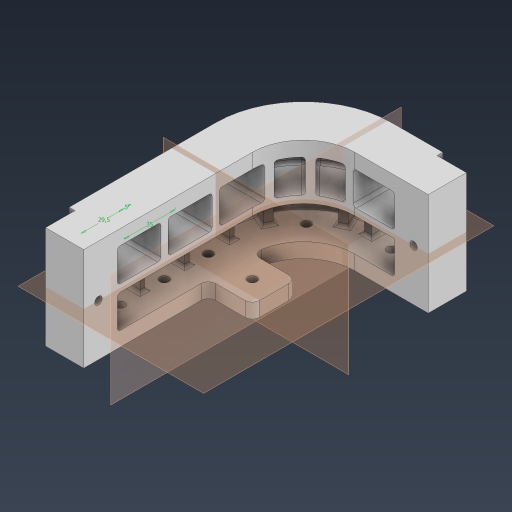
# Autodesk Inventor part: Верхняя часть столба зада
Saved by Autodesk Inventor 2023.2 (Build 272271030, 271C)
## iProperties
Created: 2025-09-30
Part Number: Верхняя часть столба зада
Material: Типовые
Document SubType Name: Modeling
Designer: Олег Коноваленко
Density: 1 g/cm^3
Appearance: По умолчанию
Author: Олег Коноваленко
Autodesk Inventor part; units mm, degrees
sketch "Эскиз1" plane through (0, 0, 0) normal (0, 1, 0) x (-1, 0, 0)
  line L0 (57.5, -90) -> (57.5, 90)
  line L1 (57.5, 90) -> (27.5, 90)
  line L2 (27.5, 90) -> (27.5, -60)
  line L3 (27.5, -60) -> (-57.5, -60)
  line L4 (-57.5, -60) -> (-57.5, -90)
  line L5 (-57.5, -90) -> (57.5, -90)
  line L6 (27.5, 90) -> (-57.5, 90) construction
  line L7 (-57.5, 90) -> (-57.5, -60) construction
  line L8 (57.5, -90) -> (-57.5, 90) construction
  line L9 (-57.5, -90) -> (57.5, 90) construction
  arc A0 (-2.5, -90) -> (57.5, -30) centre (-2.5, -30) ccw
  arc A1 (-7.5, -60) -> (27.5, -25) centre (-7.5, -25) ccw
  point P0 (0, 0)
  point P1 (0, 0)
  dimension "d0" = 115
  dimension "d1" = 180
  dimension "d2" = 30
  dimension "d3" = 30
  dimension "d5" = 70
  dimension "d6" = 60
  constraints: 20 end point, 6 perpendicular, 4 point on circle, 4 point on line, 4 tangent, 2 centre point, 1 coincident, 1 horizontal, 1 midpoint, 1 vertical
  measures "d0" distance of L4.end L0.start
  measures "d1" distance of L0.start L0.end
  measures "d2" distance of L3.end L4.end
  measures "d3" distance of L0.end L1.end
  measures "d5" diameter of A1
  measures "d6" radius of A0
extrude "Выдавливание1" add sketch "Эскиз1" along normal mid plane 70 contours A0 L5 L4 L3 L2 L1 L0 | L2 L3 A1
shell "Оболочка1" thickness 5 removed faces 3 at (-25.0806, 11.6667, -37.7869) at (24.1667, 11.6667, -60) at (-27.5, 11.6667, 13.3333)
sketch "Эскиз2" plane through (0, 0, 0) normal (0, 1, 0) x (-1, 0, 0)
  line L0 (27.5, -25) -> (27.5, 85) projected
  arc A0 (-7.5, -60) -> (27.5, -25) centre (-7.5, -25) ccw projected
  line L1 (-52.5, -60) -> (-7.5, -60) projected
  line L2 (-52.5, -85) -> (-52.5, -60) projected
  line L3 (-2.5, -85) -> (-52.5, -85) projected
  arc A1 (-2.5, -85) -> (52.5, -30) centre (-2.5, -30) ccw projected
  line L4 (52.5, 85) -> (52.5, -30) projected
  line L5 (27.5, 85) -> (52.5, 85) projected
  point P0 (0, 0)
extrude "Выдавливание2" add sketch "Эскиз2" along normal mid plane 5
ref_plane "РабПлоскость2" through (-57.5, -35, -90) normal (0, 1, 0) x (0, 0, 1)
sketch "Эскиз7" plane through (2.5, -30, -85) normal (0, 1, 0) x (1, 0, 0)
  line L0 (-30, -60) -> (-30, -170) projected
  arc A0 (5, -25) -> (-30, -60) centre (5, -60) ccw projected
  line L1 (50, -25) -> (5, -25) projected
  line L2 (50, 0) -> (50, -25) projected
  line L3 (0, 0) -> (50, 0) projected
  arc A1 (0, 0) -> (-55, -55) centre (0, -55) ccw projected
  line L4 (-55, -170) -> (-55, -55) projected
  line L5 (-30, -170) -> (-55, -170) projected
  point P0 (-2.5, -85)
extrude "Выдавливание7" add sketch "Эскиз7" along normal blind 5
mirror "Зеркальное отражение1" about plane through (0, 0, 0) normal (0, 1, 0) of "Выдавливание7"
sketch "Эскиз8" plane through (2.5, -25, -85) normal (0, 1, 0) x (1, 0, 0)
  circle A0 centre (-45, -135) radius 3.1 projected
  circle A1 centre (-45, -105) radius 3.1 projected
  circle A2 centre (-45, -75) radius 3.1 projected
  circle A3 centre (-29.2732, -23.8577) radius 3.05 projected
  circle A4 centre (15, -10) radius 3.1 projected
  point P0 (-2.5, -85)
extrude "Выдавливание8" cut sketch "Эскиз8" against normal up to next
sketch "Эскиз9" plane through (2.5, -25, -85) normal (0, 1, 0) x (1, 0, 0)
  arc A0 (5, -25) -> (-30, -60) centre (5, -60) ccw projected
  line L0 (-30, -60) -> (0, -60)
  line L1 (0, -60) -> (0, -90)
  line L2 (0, -90) -> (-30, -90)
  line L3 (-30, -90) -> (-30, -60)
  circle A1 centre (-15, -75) radius 3.1 projected
  point P0 (-2.5, -85)
  dimension "d28" = 30
  dimension "d29" = 30
  constraints: 8 end point, 2 parallel, 1 horizontal, 1 perpendicular
  measures "d28" distance of L0.start L0.end
  measures "d29" distance of L0.end L1.end
extrude "Выдавливание9" add sketch "Эскиз9" against normal blind 10
fillet "Сопряжение1" radius 5 4 edges at (-27.5, -30, 5) (2.5, -30, 5) (-27.5, -30, -25) (2.5, -30, -25)
sketch "Эскиз10" plane through (57.5, 35, -90) normal (0, 0, -1) x (-1, 0, 0)
  line L0 (0, -70) -> (50, -70) projected
  line L1 (0, 0) -> (20, 0)
  line L2 (20, 0) -> (20, -70)
  line L3 (20, -70) -> (0, -70)
  line L4 (0, -70) -> (0, 0)
  point P0 (57.5, -35)
  dimension "d33" = 20
  constraints: 8 end point, 2 parallel, 1 horizontal, 1 perpendicular, 1 point on line
  measures "d33" distance between parallel lines of L4 L2
extrude "Выдавливание10" cut sketch "Эскиз10" against normal blind 4
sketch "Эскиз11" plane through (-57.5, -35, 90) normal (-1, 0, 0) x (0, 0, 1)
  line L0 (0, 0) -> (0, 70) projected
  line L1 (0, 0) -> (-120, 0) projected
  line L2 (0, 70) -> (-20, 70)
  line L3 (-20, 70) -> (-20, 0)
  line L4 (-20, 0) -> (0, 0)
  line L5 (0, 0) -> (0, 70)
  point P0 (-90, 35)
  dimension "d36" = 20
  constraints: 8 end point, 2 parallel, 1 horizontal, 1 perpendicular, 1 point on line
  measures "d36" distance between parallel lines of L0 L3
extrude "Выдавливание11" cut sketch "Эскиз11" against normal blind 4
sketch "Эскиз12" plane through (7.5, -35, -60) normal (0, 0, 1) x (1, 0, 0)
  line L0 (0, 70) -> (50, 70) projected
  line L1 (50, 0) -> (0, 0) projected
  line L2 (50, 70) -> (27, 70)
  line L3 (27, 70) -> (27, 0)
  line L4 (27, 0) -> (50, 0)
  line L5 (50, 0) -> (50, 70)
  point P0 (-7.5, 35)
  dimension "d39" = 23
  constraints: 8 end point, 2 parallel, 1 horizontal, 1 perpendicular, 1 point on line
  measures "d39" distance between parallel lines of L5 L3
extrude "Выдавливание12" add sketch "Эскиз12" against normal up to next
sketch "Эскиз13" plane through (-27.5, -35, 90) normal (1, 0, 0) x (0, 0, -1)
  line L0 (0, 70) -> (115, 70) projected
  line L1 (80, 0) -> (0, 0) projected
  line L2 (0, 70) -> (23, 70)
  line L3 (23, 70) -> (23, 0)
  line L4 (23, 0) -> (0, 0)
  line L5 (0, 0) -> (0, 70)
  point P0 (90, 35)
  point P1 (23, 70)
  dimension "d42" = 23
  constraints: 8 end point, 2 parallel, 1 horizontal, 1 perpendicular, 1 point on line
  measures "d42" distance between parallel lines of L3 L5
extrude "Выдавливание13" add sketch "Эскиз13" against normal up to next
sketch "Эскиз14" plane through (57.5, 35, -86) normal (0, 0, -1) x (-1, 0, 0)
  circle A0 centre (10, -35) radius 2.55
  line L0 (0, -70) -> (0, 0) projected
  line L1 (-23, -35) -> (138, -35) construction
  point P0 (57.5, -35)
  dimension "d45" = 5.1
  dimension "d46" = 10
  constraints: 1 centre point, 1 point on line
  measures "d45" diameter of A0
  measures "d46" distance from line of L0 A0.centre
extrude "Выдавливание14" cut sketch "Эскиз14" against normal up to next
sketch "Эскиз15" plane through (-53.5, -35, 90) normal (-1, 0, 0) x (0, 0, 1)
  circle A0 centre (-10, 35) radius 2.55
  line L0 (0, 70) -> (0, 0) projected
  line L1 (-216, 35) -> (36, 35) construction
  point P0 (-90, 35)
  dimension "d49" = 5.1
  dimension "d50" = 10
  constraints: 1 centre point, 1 point on line
  measures "d49" diameter of A0
  measures "d50" distance from line of L0 A0.centre
extrude "Выдавливание15" cut sketch "Эскиз15" against normal up to next
sketch "Эскиз16" plane through (-52.5, 2.5, -30) normal (1, 0, 0) x (0, 0, -1)
  line L0 (-97, 0) -> (-5, 0) projected
  line L1 (-97, 22.5) -> (-5, 22.5) projected
  line L2 (-67.5, 0) -> (-62.5, 0)
  line L3 (-62.5, 0) -> (-62.5, 22.5)
  line L4 (-62.5, 22.5) -> (-67.5, 22.5)
  line L5 (-67.5, 22.5) -> (-67.5, 0)
  line L6 (-97, 0) -> (-97, 22.5) projected
  line L7 (-32.5, 0) -> (-27.5, 0)
  line L8 (-27.5, 0) -> (-27.5, 22.5)
  line L9 (-27.5, 22.5) -> (-32.5, 22.5)
  line L10 (-32.5, 22.5) -> (-32.5, 0)
  line L11 (2.5, 0) -> (7.5, 0)
  line L12 (7.5, 0) -> (7.5, 22.5)
  line L13 (7.5, 22.5) -> (2.5, 22.5)
  line L14 (2.5, 22.5) -> (2.5, 0)
  point P0 (-30, -2.5)
  point P1 (-6.5, 22.5)
  point P2 (-6.5, 0)
  point P3 (-27.5, 0)
  point P4 (-27.5, 22.5)
  dimension "d53" = 5
  dimension "d54" = 29.5
  dimension "d57" = 35
  constraints: 24 end point, 2 horizontal, 2 parallel, 2 point on line, 1 perpendicular, 16 other
  measures "d53" distance between parallel lines of L5 L3
  measures "d54" distance between parallel lines of L6 L5
  measures "d57" distance of L2.start L7.start
extrude "Выдавливание16" add sketch "Эскиз16" along normal up to surface (25 mm away) contours L5 L1 L3 L0 | L10 L1 L8 L0
extrude "Выдавливание17" add sketch "Эскиз16" along normal up to surface contours L14 L13 L12 L11 round surface about axis through (7.5, 0, -25) along (0, 1, 0) radius 35 far side no
sketch "Эскиз17" plane through (2.5, 2.5, -85) normal (0, 0, 1) x (1, 0, 0)
  line L0 (5, 22.5) -> (32, 22.5) projected
  line L1 (5, 0) -> (32, 0) projected
  line L2 (-1, 22.5) -> (4, 22.5)
  line L3 (4, 22.5) -> (4, 0)
  line L4 (4, 0) -> (-1, 0)
  line L5 (-1, 0) -> (-1, 22.5)
  line L6 (32, 22.5) -> (32, 0) projected
  point P0 (-2.5, -2.5)
  dimension "d66" = 5
  dimension "d67" = 33
  constraints: 8 end point, 2 parallel, 2 point on line, 1 horizontal, 1 perpendicular
  measures "d66" distance between parallel lines of L3 L5
  measures "d67" distance between parallel lines of L6 L5
extrude "Выдавливание18" add sketch "Эскиз17" along normal up to surface round surface about axis through (7.5, 0, -25) along (0, 1, 0) radius 35 far side no
sketch "Эскиз18" plane through (0, 2.5, 0) normal (0, 1, 0) x (1, 0, 0)
  line L0 (-16.6252, 50.357) -> (-35.7701, 69.5019)
  arc A0 (1.5, 84.9909) -> (-51.9862, 37.5) centre (2.5, 30) ccw projected
  line L1 (-32.0172, 72.8201) -> (-12.7466, 53.5495)
  arc A1 (1.5, 59.4819) -> (-25.1917, 37.5) centre (7.5, 25) ccw projected
  line L2 (1.5, 59.4819) -> (1.5, 84.9909) projected
  line L3 (-26.1976, 59.9294) -> (-22.6621, 63.465) construction
  line L4 (-24.4299, 61.6972) -> (-14.75, 52.0173) construction
  point P0 (0, 0)
  dimension "d70" = 5
  dimension "d71" = 45
  constraints: 8 end point, 5 point on circle, 2 midpoint, 2 perpendicular, 1 parallel, 1 point on line
  measures "d70" distance between parallel lines of L1 L0
  measures "d71" angle of L2 L1
extrude "Выдавливание19" add sketch "Эскиз18" along normal up to next contours L0 A0 L1 A1
sketch "Эскиз19" plane through (-52.5, -25, -30) normal (1, 0, 0) x (0, 0, -1)
  line L0 (0, 22.5) -> (-97, 22.5) projected
  line L1 (-97, 0) -> (0, 0) projected
  line L2 (-66.5, 22.5) -> (-63.5, 22.5)
  line L3 (-63.5, 22.5) -> (-63.5, 0)
  line L4 (-63.5, 0) -> (-66.5, 0)
  line L5 (-66.5, 0) -> (-66.5, 22.5)
  line L6 (-97, 0) -> (-97, 22.5) projected
  line L7 (-36, 22.5) -> (-33, 22.5)
  line L8 (-33, 22.5) -> (-33, 0)
  line L9 (-33, 0) -> (-36, 0)
  line L10 (-36, 0) -> (-36, 22.5)
  line L11 (-5.5, 22.5) -> (-2.5, 22.5)
  line L12 (-2.5, 22.5) -> (-2.5, 0)
  line L13 (-2.5, 0) -> (-5.5, 0)
  line L14 (-5.5, 0) -> (-5.5, 22.5)
  point P0 (-30, 25)
  point P1 (-5.5, 0)
  point P2 (-36, 22.5)
  point P3 (-36, 0)
  point P4 (-66.5, 0)
  dimension "d74" = 3
  dimension "d75" = 30.5
  dimension "d85" = 30.5
  constraints: 24 end point, 2 horizontal, 2 parallel, 2 point on line, 1 perpendicular, 16 other
  measures "d74" distance between parallel lines of L3 L5
  measures "d75" distance between parallel lines of L6 L5
  measures "d85" distance of L2.start L7.start
extrude "Выдавливание20" add sketch "Эскиз19" along normal blind 10 contours L12 L1 L14 L0 | L8 L1 L10 L0 | L3 L1 L5 L0
sketch "Эскиз20" plane through (2.5, -25, -85) normal (0, 0, 1) x (1, 0, 0)
  line L0 (32, 22.5) -> (5, 22.5) projected
  line L1 (5, 0) -> (32, 0) projected
  line L2 (-3.5, 22.5) -> (1.5, 22.5)
  line L3 (1.5, 22.5) -> (1.5, 0)
  line L4 (1.5, 0) -> (-3.5, 0)
  line L5 (-3.5, 0) -> (-3.5, 22.5)
  line L6 (32, 22.5) -> (32, 0) projected
  point P0 (-2.5, 25)
  dimension "d92" = 5
  dimension "d93" = 30.5
  constraints: 8 end point, 2 parallel, 2 point on line, 1 horizontal, 1 perpendicular
  measures "d92" distance between parallel lines of L3 L5
  measures "d93" distance between parallel lines of L6 L3
extrude "Выдавливание21" add sketch "Эскиз20" along normal blind 10
sketch "Эскиз21" plane through (2.5, -25, -85) normal (0, 1, 0) x (1, 0, 0)
  arc A0 (-3.5, -0.1115) -> (-55, -55) centre (0, -55) ccw projected
  line L0 (-51.4576, -35.5805) -> (-42.5304, -39.7433)
  line L1 (-42.5304, -39.7433) -> (-40.4173, -35.2117)
  line L2 (-40.4173, -35.2117) -> (-49.4804, -30.9856)
  line L3 (-21.7558, -4.4858) -> (-17.3702, -13.8905)
  line L4 (-17.3702, -13.8905) -> (-12.8387, -11.7774)
  line L5 (-12.8387, -11.7774) -> (-17.0649, -2.7143)
  line L6 (-55, -57.5) -> (-45, -57.5) projected
  line L7 (-3.5, -10) -> (-3.5, -0.1115) projected
  circle A1 centre (-29.2732, -23.8577) radius 3.05 projected
  point P0 (-2.5, -85)
  point P1 (-3.5, -26.0478)
  dimension "d96" = 5
  dimension "d97" = 5
  dimension "d98" = 25
  dimension "d99" = 25
  dimension "d100" = 10
  dimension "d101" = 10
  dimension "d102" = 15
  dimension "d103" = 15
  constraints: 12 end point, 4 perpendicular, 4 point on circle
  measures "d96" distance between parallel lines of L0 L2
  measures "d97" distance between parallel lines of L5 L3
  measures "d98" angle of L6 L0
  measures "d99" angle of L7 L5
  measures "d100" distance from line of L1 L2.end
  measures "d101" distance from line of L4 L5.end
  measures "d102" distance from line of L3 A1.centre
  measures "d103" distance from line of A1.centre L2
extrude "Выдавливание22" add sketch "Эскиз21" along normal up to next contours L5 L4 L3 A0 | L2 L1 L0 A0
fillet "Сопряжение2" radius 2 50 edges at (-52.5, 2.5, 52.25) (-52.5, 13.75, 67) (-52.5, 25, 52.25) (-52.5, 13.75, 37.5) (-40, 25, 37.5) (-40, 25, 67) (-40, 2.5, 67) (-40, 2.5, 37.5) (-52.5, 13.75, 32.5) (-52.5, 2.5, 17.5) (-40, 2.5, 32.5) (-52.5, 25, 17.5) (-40, 25, 32.5) (-40, 25, 2.5) (-52.5, 13.75, 2.5) (-40, 2.5, 2.5) (-52.4858, 2.5, -31.2503) (-52.5, 2.5, -16.25) (-52.4432, 13.75, -32.5) (-39.5651, 2.5, -32.5) (-40, 2.5, -2.5) (-52.5, 13.75, -2.5) (-52.4858, 25, -31.2503) (-52.5, 25, -16.25) (-40, 25, -2.5) (-39.5651, 25, -32.5) (-51.9862, 13.75, -37.5) (-38.589, 25, -37.5) (-46.5608, 25, -54.8603) (-26.1976, 25, -59.9294) (-35.7701, 13.75, -69.5019) (-26.1976, 2.5, -59.9294) (-46.5608, 2.5, -54.8603) (-38.589, 2.5, -37.5) (-22.3819, 2.5, -63.1848) (-16.2723, 2.5, -81.6972) (-32.0172, 13.75, -72.8201) (-16.2723, 25, -81.6972) (-22.3819, 25, -63.1848) (1.5, 13.75, -84.9909) (1.5, 2.5, -72.2364) (1.5, 25, -72.2364) (6.5, 2.5, -72.4929) (20.5, 2.5, -85) (6.5, 13.75, -85) (20.5, 25, -85) (6.5, 25, -72.4929) (34.5, 13.75, -85) (34.5, 25, -72.5) (34.5, 2.5, -72.5)
fillet "Сопряжение3" radius 2 50 edges at (34.5, -25, -72.5) (34.5, -13.75, -85) (19.25, -2.5, -85) (4, -13.75, -85) (4, -25, -80) (1.5, -25, -75) (1.5, -2.5, -75) (4, -2.5, -80) (-1, -13.75, -84.8885) (-1, -2.5, -79.9443) (-1, -25, -79.9443) (-7.8645, -25, -84.0146) (-12.4518, -25, -77.7541) (-14.5649, -13.75, -82.2857) (-12.6045, -25, -72.166) (-12.4518, -2.5, -77.7541) (-7.8645, -2.5, -84.0146) (-17.063, -2.5, -75.8119) (-12.6045, -2.5, -72.166) (-19.2558, -13.75, -80.5142) (-17.063, -25, -75.8119) (-35.5027, -2.5, -69.7592) (-46.9804, -13.75, -54.0144) (-42.4488, -25, -51.9013) (-38.9738, -25, -47.5225) (-42.4488, -2.5, -51.9013) (-38.9738, -2.5, -47.5225) (-48.9576, -13.75, -49.4195) (-52.5, -2.5, -28.75) (-51.6071, -2.5, -39.87) (-44.494, -2.5, -47.3381) (-52.5, -25, -28.75) (-51.6071, -25, -39.87) (-44.494, -25, -47.3381) (-47.5, -25, -27.5) (-52.5, -13.75, -27.5) (-42.5, -25, -26) (-47.5, -25, -24.5) (-52.5, -13.75, -24.5) (-47.5, -2.5, -27.5) (-47.5, -2.5, -24.5) (-52.5, -2.5, -10.75) (-52.5, -2.5, 19.75) (-52.5, -2.5, 51.75) (-47.5, -2.5, 36.5) (-42.5, -2.5, 35) (-42.5, -2.5, 4.5) (-47.5, -2.5, 6) (-42.5, -2.5, -26) (-52.5, -13.75, 36.5)
fillet "Сопряжение4" radius 2 20 edges at (-51.9142, -3.0858, 3) (-52.5, -14.75, 3) (-41.5, -2.5, 3) (-46.5, -2.5, 3) (-47.5, -25, 3) (-47.5, -25, 6) (-42.5, -25, 4.5) (-51.9142, -3.0858, 33.5) (-52.5, -14.75, 33.5) (-41.5, -2.5, 33.5) (-46.5, -2.5, 33.5) (-47.5, -25, 33.5) (-52.5, -25, 19.75) (-52.5, -25, -9.75) (-46.5, -25, 36.5) (-42.5, -25, 35) (-51.9142, -3.0858, 67) (-52.5, -14.75, 67) (-39, -2.5, 67) (-40, -25, 67)
fillet "Сопряжение5" radius 2 3 edges at (-51.9142, -3.0858, 6.5858) (-51.9142, -24.4142, 6.5858) (-52.5, -13.75, 6)
